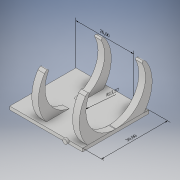
# Autodesk Inventor part: FanGrasp
Saved by Autodesk Inventor 2019 (Build 230136000, 136)
## iProperties
Created: 2018-06-07
Part Number: FanGrasp
Material: Ogólny
Document SubType Name: Modeling
Designer: Kamil
Density: 1 g/cm^3
Appearance: Domyślna
Author: Kamil
Autodesk Inventor part; units mm, degrees
sketch "Szkic1" plane through (0, 0, 0) normal (0, 1, 0) x (-1, 0, 0)
  line L0 (-16.5, 15) -> (16.5, 15)
  line L1 (16.5, 15) -> (16.5, -15)
  line L2 (16.5, -15) -> (-16.5, -15)
  line L3 (-16.5, -15) -> (-16.5, 15)
  line L4 (-16.5, 15) -> (16.5, -15) construction
  line L5 (16.5, 15) -> (-16.5, -15) construction
  point P0 (0, 0)
  dimension "d0" = 33
  dimension "d1" = 30
  constraints: 12 end point, 2 midpoint, 2 parallel, 1 horizontal, 1 perpendicular
  measures "d0" distance of L1.end L2.end
  measures "d1" distance of L0.end L1.end
extrude "Wyciągnięcie proste1" add sketch "Szkic1" along normal blind 1.5
sketch "Szkic2" plane through (-16.5, 0, 15) normal (0, 0, 1) x (1, 0, 0)
  circle A0 centre (26, 1) radius 1
  point P0 (16.5, 0)
  dimension "d4" = 2
  constraints: 1 centre point
  measures "d4" diameter of A0
sketch "Szkic3" plane through (16.5, 0, -15) normal (0, 0, -1) x (-1, 0, 0)
  circle A0 centre (7, 1) radius 1
  point P0 (16.5, 0)
  dimension "d5" = 2
  constraints: 1 centre point
  measures "d5" diameter of A0
extrude "Wyciągnięcie proste2" add sketch "Szkic3" along normal blind 1
extrude "Wyciągnięcie proste3" add sketch "Szkic2" along normal blind 1
sketch "Szkic4" plane through (16.5, 0, 15) normal (1, 0, 0) x (0, 0, -1)
  arc A0 (3.456604, 22) -> (15, 1.5) centre (15, 15) ccw
  line L0 (1.875595, 22) -> (3.456604, 22)
  line L1 (26.543396, 22) -> (28.124405, 22)
  arc A1 (1.875595, 22) -> (2.270166, 1.502318) centre (15, 12) ccw
  line L2 (2.270166, 1.502318) -> (14.821882, 1.501175)
  line L3 (15.17566, 1.501143) -> (27.727922, 1.5)
  line L4 (14.821882, 1.501175) -> (15.17566, 1.501143)
  arc A2 (2.270166, 1.502318) -> (2.272078, 1.5) centre (15, 12) ccw
  arc A3 (15, 1.5) -> (26.543396, 22) centre (15, 15) ccw
  arc A4 (27.727922, 1.5) -> (28.124405, 22) centre (15, 12) ccw
  point P0 (15, 0)
  constraints: 14 point on circle, 10 end point, 5 centre point, 2 horizontal
sketch "Szkic4 outline for Wyciągnięcie proste4" plane through (16.5, 0, 15) normal (1, 0, 0) x (0, 0, -1)
  line L0 (3.456604, 22) -> (1.875595, 22)
  arc A0 (14.821882, 1.501175) -> (3.456604, 22) centre (15, 15) cw
  line L1 (2.270166, 1.502318) -> (14.821882, 1.501175)
  arc A1 (1.875595, 22) -> (2.270166, 1.502318) centre (15, 12) ccw
  arc A2 (26.543396, 22) -> (15.17566, 1.501143) centre (15, 15) cw
  line L2 (28.124405, 22) -> (26.543396, 22)
  arc A3 (27.727922, 1.5) -> (28.124405, 22) centre (15, 12) ccw
  line L3 (15.17566, 1.501143) -> (27.727922, 1.5)
extrude "Wyciągnięcie proste4" add sketch "Szkic4 outline for Wyciągnięcie proste4" against normal blind 3
ref_plane "Płaszczyzna konstrukcyjna1" through (-11.5, 3.25, -15) normal (-1, 0, 0) x (0, 0, 1)
ref_plane "Płaszczyzna konstrukcyjna2" through (-11.5, -0.25, -15) normal (-1, 0, 0) x (0, 0, 1)
ref_plane "Płaszczyzna konstrukcyjna3" through (-5, -0.25, -15) normal (-1, 0, 0) x (0, 0, 1)
sketch "Szkic5" plane through (-5, -0.25, -15) normal (-1, 0, 0) x (0, 0, 1)
  arc A0 (3.456604, 22) -> (15, 1.5) centre (15, 15) ccw
  line L0 (1.875595, 22) -> (3.456604, 22)
  line L1 (26.543396, 22) -> (28.124405, 22)
  arc A1 (1.875595, 22) -> (2.270166, 1.502318) centre (15, 12) ccw
  line L2 (2.270166, 1.502318) -> (14.821882, 1.501175)
  line L3 (15.17566, 1.501143) -> (27.727922, 1.5)
  line L4 (14.821882, 1.501175) -> (15.17566, 1.501143)
  arc A2 (2.270166, 1.502318) -> (2.272078, 1.5) centre (15, 12) ccw
  arc A3 (15, 1.5) -> (26.543396, 22) centre (15, 15) ccw
  arc A4 (27.727922, 1.5) -> (28.124405, 22) centre (15, 12) ccw
  point P0 (15, 0)
  constraints: 14 point on circle, 10 end point, 5 centre point, 2 horizontal
extrude "Wyciągnięcie proste5" add sketch "Szkic5" against normal blind 3
fillet "Zaokrąglenie1" radius 2 1 edges at (15, 22, 13.1244)
fillet "Zaokrąglenie2" radius 2 1 edges at (15, 22, -13.1244)
fillet "Zaokrąglenie3" radius 2 1 edges at (-3.5, 21.75, -13.1244)
fillet "Zaokrąglenie4" radius 2 1 edges at (-3.5, 21.75, 13.1244)
fillet "Zaokrąglenie5" radius 0.5 1 edges at (15, 22, 11.5434)
fillet "Zaokrąglenie6" radius 0.5 1 edges at (-3.5, 21.75, 11.5434)
fillet "Zaokrąglenie7" radius 0.5 1 edges at (-3.5, 21.75, -11.5434)
fillet "Zaokrąglenie8" radius 0.5 1 edges at (15, 22, -11.5434)
